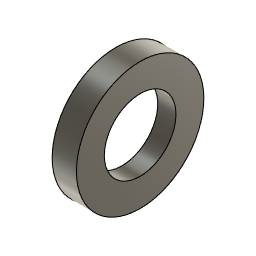
轴承套 v1 (Autodesk Fusion 360 design; units mm, degrees)
Autodesk Fusion 360 part; units mm, degrees
sketch "草图1" plane through (0, 0, 0) normal (1, 0, 0) x (0, 1, 0)
  circle A0 centre (0, 0) radius 5.9
  circle A1 centre (0, 0) radius 8
  circle A2 centre (0, 0) radius 6.75
  circle A3 centre (0, 0) radius 10.5
  dimension "d1" = 11.8
  dimension "d2" = 16
  dimension "d3" = 13.5
  dimension "d6" = 21
  constraint coincident A0.centre A1.centre
  constraint concentric A0 A1
  constraint concentric A1 A2
  constraint concentric A1 A3
  measures "d1" diameter of A0
  measures "d2" diameter of A1
  measures "d3" diameter of A2
  measures "d6" diameter of A3
extrude "拉伸1" add sketch "草图1" along normal blind 3 contours A1 | A2
extrude "拉伸2" add sketch "草图1" along normal blind 3 and the other way blind 1 contours A3
